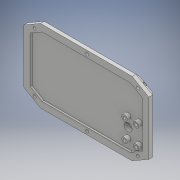
# Autodesk Inventor part: Topv5
Saved by Autodesk Inventor 2017 (Build 210142000, 142)
## iProperties
Created: 2020-03-10
Part Number: Topv5
Material: Generic
Document SubType Name: Modeling
Designer: Manny
Density: 1 g/cm^3
Appearance: Default
Author: Manny
Autodesk Inventor part; units mm, degrees
ref_plane "YZ Plane" through (0, 0, 0) normal (1, 0, 0) x (0, 1, 0)
ref_plane "XZ Plane" through (0, 0, 0) normal (0, 1, 0) x (-1, 0, 0)
sketch "Sketch5" plane through (0, 0, 0) normal (0, 1, 0) x (-1, 0, 0)
  line L0 (0, 0) -> (-95, 0)
  line L1 (-95, 0) -> (-95, -65)
  line L2 (-95, -65) -> (0, -65)
  line L3 (0, -65) -> (0, 0)
  line L4 (0, -65) -> (12.9904, -57.5)
  line L5 (12.9904, -57.5) -> (12.9904, -7.5)
  line L6 (12.9904, -7.5) -> (0, 0)
  line L7 (-95, -65) -> (-107.9904, -57.5)
  line L8 (-107.9904, -57.5) -> (-107.9904, -7.5)
  line L9 (-107.9904, -7.5) -> (-95, 0)
  dimension "d23" = 95
  dimension "d24" = 65
  dimension "d25" = 15
  dimension "d26" = 15
  dimension "d27" = 120
  dimension "d28" = 15
  dimension "d29" = 15
  dimension "d30" = 120
  constraints: 20 end point, 2 parallel, 2 vertical, 1 horizontal, 1 perpendicular
  measures "d23" distance of L0.start L0.end
  measures "d24" distance of L2.end L0.start
  measures "d25" distance of L2.end L4.end
  measures "d26" distance of L5.end L0.start
  measures "d27" angle of L5 L4
  measures "d28" distance of L1.end L7.end
  measures "d29" distance of L8.end L0.end
  measures "d30" angle of L8 L9
extrude "Extrusion3" add sketch "Sketch5" along normal blind 8
sketch "Sketch6" plane through (0, 0, 0) normal (0, -1, 0) x (1, 0, 0)
  line L0 (0, 7) -> (87, 7)
  line L1 (95, -72) -> (8, -72)
  line L2 (0, 0) -> (95, 0) projected
  line L3 (95, -65) -> (0, -65) projected
  line L4 (96.8756, 7) -> (114.9904, -3.4585)
  line L5 (95, 0) -> (107.9904, -7.5) projected
  line L6 (114.9904, -3.4585) -> (114.9904, -61.5415)
  line L7 (107.9904, -7.5) -> (107.9904, -57.5) projected
  line L8 (96.8756, -72) -> (114.9904, -61.5415)
  line L9 (107.9904, -57.5) -> (95, -65) projected
  line L10 (107.9904, -57.5) -> (95, -65) projected
  line L11 (87, 7) -> (96.8756, 7)
  line L12 (95, -72) -> (96.8756, -72)
  line L13 (0, 7) -> (-1.8756, 7)
  line L14 (-19.9904, -3.4585) -> (-1.8756, 7)
  line L15 (-19.9904, -61.5415) -> (-2.8038, -71.4641)
  line L16 (0, -65) -> (-12.9904, -57.5) projected
  line L17 (-12.9904, -7.5) -> (0, 0) projected
  line L18 (-19.9904, -61.5415) -> (-19.9904, -3.4585)
  line L19 (-12.9904, -57.5) -> (-12.9904, -7.5) projected
  line L20 (0, -65) -> (-12.9904, -57.5) projected
  line L21 (-12.9904, -7.5) -> (-12.9904, -57.5)
  line L22 (-12.9904, -57.5) -> (0, -65)
  line L23 (95, -65) -> (0, -65) projected
  line L24 (0, -65) -> (95, -65)
  line L25 (95, -65) -> (107.9904, -57.5)
  line L26 (107.9904, -7.5) -> (107.9904, -57.5)
  line L27 (95, 0) -> (107.9904, -7.5) projected
  line L28 (107.9904, -7.5) -> (95, 0)
  line L29 (0, 0) -> (-12.9904, -7.5)
  line L30 (95, 0) -> (0, 0)
  line L31 (8, -72) -> (-1.8756, -72)
  line L32 (-2.8038, -71.4641) -> (-1.8756, -72)
  dimension "d33" = 7
  dimension "d34" = 7
  dimension "d35" = 7
  dimension "d36" = 7
  dimension "d37" = 7
  dimension "d38" = 7
  dimension "d39" = 7
  dimension "d40" = 7
  constraints: 44 end point, 8 parallel, 5 collinear, 5 horizontal, 3 vertical, 2 point on line, 1 perpendicular
  measures "d33" distance between parallel lines of L2 L0
  measures "d34" distance between parallel lines of L1 L3
  measures "d35" distance between parallel lines of L5 L4
  measures "d36" distance between parallel lines of L6 L7
  measures "d37" distance between parallel lines of L9 L8
  measures "d38" distance between parallel lines of L17 L14
  measures "d39" distance between parallel lines of L16 L15
  measures "d40" distance between parallel lines of L19 L18
extrude "Extrusion4" add sketch "Sketch6" along normal blind 2 and the other way blind 8
chamfer "Chamfer1" distance 6 angle 45 8 edges at (47.5, 8, 7) (-10.933, 8, 1.7707) (-19.9904, 8, -32.5) (-10.933, 8, -66.7707) (47.5, 8, -72) (105.933, 8, -66.7707) (114.9904, 8, -32.5) (105.933, 8, 1.7707)
sketch "Sketch7" plane through (0, 0, 0) normal (0, -1, 0) x (1, 0, 0)
  line L0 (86.4904, -40.25) -> (94.9904, -40.25)
  line L1 (94.9904, -40.25) -> (94.9904, -48.75)
  line L2 (94.9904, -48.75) -> (86.4904, -48.75)
  line L3 (86.4904, -48.75) -> (86.4904, -40.25)
  line L4 (96.8756, 7) -> (-1.8756, 7) projected
  line L5 (114.9904, -61.5415) -> (114.9904, -3.4585) projected
  circle A0 centre (90.7404, -55) radius 3
  circle A1 centre (90.7404, -34) radius 3
  circle A2 centre (103.1404, -34) radius 3
  circle A3 centre (103.1404, -55) radius 3
  circle A4 centre (90.7404, -44.5) radius 4.25
  circle A5 centre (46.5, 2.8174) radius 1.834
  circle A6 centre (46.5, -64.297) radius 1.834
  line L6 (-1.8756, -72) -> (96.8756, -72) projected
  point P0 (0, 0)
  dimension "d48" = 8.5
  dimension "d50" = 20
  dimension "d51" = 6.25
  dimension "d52" = 8.15
  dimension "d53" = 12.4
  dimension "d54" = 0
  dimension "d55" = 21
  dimension "d56" = 12.4
  dimension "d57" = 0
  dimension "d58" = 0
  dimension "d59" = 6
  dimension "d61" = 8.5
  dimension "d107" = 27.5
  constraints: 8 end point, 7 centre point, 3 equal radius, 2 parallel, 2 perpendicular, 2 tangent, 1 horizontal
  measures "d48" distance of L0.end L1.end
  measures "d50" distance between parallel lines of L5 L1
  measures "d51" distance from line of L2 A0.centre
  measures "d52" distance from line of L1 A3.centre
  measures "d53" distance of A0.centre A3.centre
  measures "d54" vertical distance of A0.centre A3.centre
  measures "d55" distance of A1.centre A0.centre
  measures "d56" distance of A2.centre A1.centre
  measures "d57" vertical distance of A1.centre A2.centre
  measures "d58" horizontal distance of A3.centre A2.centre
  measures "d59" diameter of A3
  measures "d61" diameter of A4
  measures "d107" distance from line of L6 A4.centre
sketch "Sketch9" plane through (0, -2, 0) normal (0, -1, 0) x (1, 0, 0)
  circle A0 centre (-8.2452, -0.7189) radius 1.6
  line L0 (0, -65) -> (-12.9904, -57.5) projected
  line L1 (0, -65) -> (-1.8756, -72) projected
  line L2 (95, -65) -> (0, -65) projected
  line L3 (107.9904, -7.5) -> (107.9904, -57.5) projected
  line L4 (0, 0) -> (95, 0) projected
  line L5 (-12.9904, -7.5) -> (-16.4904, -1.4378)
  line L6 (-19.9904, -3.4585) -> (-1.8756, 7) projected
  line L7 (0, 0) -> (-3.5, 6.0622)
  line L8 (-12.9904, -57.5) -> (-19.9904, -61.5415) projected
  line L9 (-12.9904, -57.5) -> (-15.4904, -61.8301)
  line L10 (0, -65) -> (-2.5, -69.3301)
  line L11 (95, -65) -> (97.5, -69.3301)
  line L12 (95, 0) -> (98.5, 6.0622)
  line L13 (96.8756, 7) -> (114.9904, -3.4585) projected
  line L14 (107.9904, -7.5) -> (114.9904, -3.4585) projected
  line L15 (107.9904, -7.5) -> (111.4904, -1.4378)
  line L16 (107.9904, -57.5) -> (111.4904, -63.5622)
  line L17 (96.8756, -72) -> (114.9904, -61.5415) projected
  line L18 (107.9904, -57.5) -> (95, -65) projected
  line L19 (95, 0) -> (107.9904, -7.5) projected
  circle A1 centre (-8.2452, -64.2811) radius 1.6
  circle A2 centre (103.2452, -64.2811) radius 1.6
  circle A3 centre (103.2452, -0.7189) radius 1.6
  circle A4 centre (48.5, 3.5) radius 1.6
  circle A5 centre (48.5, -68.5) radius 1.6
  line L20 (95, -65) -> (95, -72)
  line L21 (-1.8756, -72) -> (96.8756, -72) projected
  line L22 (95, 0) -> (95, 7)
  line L23 (96.8756, 7) -> (-1.8756, 7) projected
  dimension "d62" = 90
  dimension "d63" = 90
  dimension "d64" = 90
  dimension "d65" = 7.5
  dimension "d66" = 3.5
  dimension "d67" = 3.2
  dimension "d68" = 7.5
  dimension "d69" = 3.5
  dimension "d70" = 3.5
  dimension "d71" = 7.5
  dimension "d72" = 7.5
  dimension "d73" = 3.5
  dimension "d76" = 3.5
  dimension "d77" = 46.5
  dimension "d78" = 3.5
  dimension "d79" = 46.5
  constraints: 20 end point, 8 point on line, 6 centre point, 5 equal radius, 4 coincident, 4 parallel, 1 perpendicular, 1 vertical
  measures "d62" angle of L18 L16
  measures "d63" angle of L18 L11
  measures "d64" angle of L19 L12
  measures "d65" distance from line of L5 A0.centre
  measures "d66" distance from line of L6 A0.centre
  measures "d67" diameter of A0
  measures "d68" distance from line of L10 A1.centre
  measures "d69" distance from line of L0 A1.centre
  measures "d70" distance from line of L18 A2.centre
  measures "d71" distance from line of L11 A2.centre
  measures "d72" distance from line of L12 A3.centre
  measures "d73" distance from line of L19 A3.centre
  measures "d76" distance from line of L4 A4.centre
  measures "d77" distance from line of L22 A4.centre
  measures "d78" distance from line of L2 A5.centre
  measures "d79" distance from line of L20 A5.centre
extrude "Extrusion6" cut sketch "Sketch9" against normal blind 2.5 contours A0 | A1 | A2 | A3 | A4 | A5
sketch "Sketch13" plane through (48.5, 0.5, 3.5) normal (0, -1, 0) x (1, 0, 0)
  circle A0 centre (0, 0) radius 2
  circle A1 centre (54.7452, -4.2189) radius 2
  circle A2 centre (54.7452, -67.7811) radius 2
  circle A3 centre (0, -72) radius 2
  circle A4 centre (-56.7452, -67.7811) radius 2
  circle A5 centre (-56.7452, -4.2189) radius 2
  circle A6 centre (-56.7452, -4.2189) radius 1.6 projected
  circle A7 centre (0, 0) radius 1.6 projected
  circle A8 centre (54.7452, -4.2189) radius 1.6 projected
  circle A9 centre (54.7452, -67.7811) radius 1.6 projected
  circle A10 centre (0, -72) radius 1.6 projected
  circle A11 centre (-56.7452, -67.7811) radius 1.6 projected
  point P0 (-48.5, -3.5)
  dimension "d90" = 4
  dimension "d91" = 4
  dimension "d92" = 4
  dimension "d93" = 4
  dimension "d94" = 4
  dimension "d95" = 4
  constraints: 6 centre point, 6 concentric
  measures "d90" diameter of A5
  measures "d91" diameter of A0
  measures "d92" diameter of A3
  measures "d93" diameter of A4
  measures "d94" diameter of A2
  measures "d95" diameter of A1
extrude "Extrusion7" cut sketch "Sketch13" against normal blind 10 contours A0 | A1 | A2 | A3 | A4 | A5 | A6 | A7 | A8 | A9 | A10 | A11
extrude "Extrusion8" add sketch "Sketch7" along normal blind 4 contours A0 | A1 | A2 | A3
sketch "Sketch14" plane through (0, 0, 0) normal (0, -1, 0) x (1, 0, 0)
  line L0 (86.4904, -48.75) -> (94.9904, -48.75)
  line L1 (94.9904, -48.75) -> (94.9904, -40.25)
  line L2 (94.9904, -40.25) -> (86.4904, -40.25)
  line L3 (86.4904, -40.25) -> (86.4904, -48.75)
  line L4 (95, -65) -> (0, -65) projected
  line L5 (107.9904, -7.5) -> (107.9904, -57.5) projected
  circle A0 centre (90.7404, -44.5) radius 4.25
  circle A1 centre (90.7404, -55) radius 3 projected
  point P0 (0, 0)
  dimension "d100" = 8.5
  dimension "d101" = 8.5
  dimension "d103" = 13
  dimension "d104" = 8.5
  dimension "d108" = 9.25
  constraints: 8 end point, 2 parallel, 2 tangent, 1 centre point, 1 horizontal, 1 perpendicular
  measures "d100" distance of L0.start L0.end
  measures "d101" distance of L0.end L1.end
  measures "d103" distance between parallel lines of L5 L1
  measures "d104" diameter of A0
extrude "Extrusion9" cut sketch "Sketch14" against normal blind 10 contours A0
ref_plane "Work Plane1" through (0, -6, 0) normal (0, -1, 0) x (1, 0, 0)
sketch "Sketch15" plane through (90.7404, -4, -34) normal (0, -1, 0) x (1, 0, 0)
  circle A0 centre (0, 0) radius 1.6
  circle A1 centre (12.4, 0) radius 1.6
  line L0 (12.4, 0) -> (0, 0)
  line L1 (0, 0) -> (0, -21)
  line L2 (0, -21) -> (12.4, -21)
  line L3 (12.4, -21) -> (12.4, 0)
  circle A2 centre (12.4, -21) radius 1.6
  circle A3 centre (0, -21) radius 1.6
  point P0 (-90.7404, 34)
  dimension "d110" = 3.2
  dimension "d111" = 3.2
  dimension "d112" = 12.4
  dimension "d113" = 21
  dimension "d114" = 3.2
  dimension "d115" = 3.2
  constraints: 8 end point, 4 centre point, 2 coincident, 2 parallel, 1 horizontal, 1 perpendicular
  measures "d110" diameter of A0
  measures "d111" diameter of A1
  measures "d112" distance of L0.start L0.end
  measures "d113" distance of L0.end L1.end
  measures "d114" diameter of A2
  measures "d115" diameter of A3
extrude "Extrusion10" cut sketch "Sketch15" against normal blind 2.5 contours L0 L1 A0 | A0 L1 L0 | L0 L3 A1 | A1 L3 L0 | A3 L2 L1 | L1 L2 A3 | A2 L2 L3 | L3 L2 A2
sketch "Sketch16" plane through (0, 8, 0) normal (0, 1, 0) x (1, 0, 0)
  circle A0 centre (90.7404, 44.5) radius 5
  circle A1 centre (90.7404, 44.5) radius 4.25 projected
  point P0 (0, 0)
  dimension "d118" = 10
  constraints: 1 centre point, 1 concentric
  measures "d118" diameter of A0
extrude "Extrusion11" cut sketch "Sketch16" against normal blind 3.175
body "Solid2"
